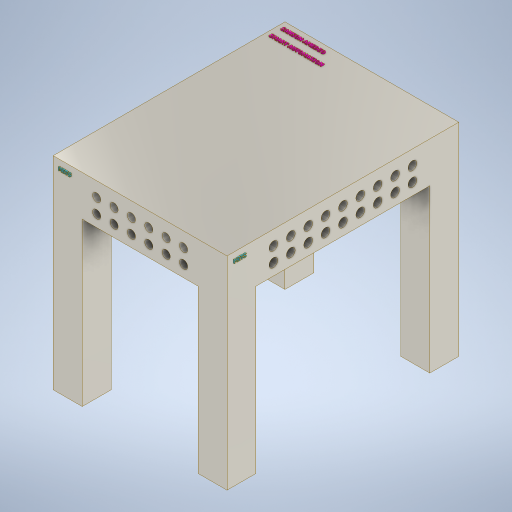
# Autodesk Inventor part: tavola d'appoggio 03-06-2023
Saved by Autodesk Inventor 2023 (Build 270158000, 158)
## iProperties
Created: 2023-03-06
Part Number: tavola d'appoggio 03-06-2023
Material: Generico
Document SubType Name: Modeling
Designer: Admin
Density: 1 g/cm^3
Appearance: Titanio
Author: Admin
Autodesk Inventor part; units mm, degrees
ref_plane "YZ Plane" through (0, 0, 0) normal (1, 0, 0) x (0, 1, 0)
ref_plane "XZ Plane" through (0, 0, 0) normal (0, 1, 0) x (-1, 0, 0)
ref_plane "XY Plane" through (0, 0, 0) normal (0, 0, 1) x (1, 0, 0)
sketch "Schizzo1" plane through (0, 0, 0) normal (0, 1, 0) x (-1, 0, 0)
  line L0 (150, 200) -> (-150, 200)
  line L1 (-150, 200) -> (-150, -200)
  line L2 (-150, -200) -> (150, -200)
  line L3 (150, -200) -> (150, 200)
  line L4 (150, 200) -> (100, 200)
  line L5 (100, 200) -> (100, 150)
  line L6 (100, 150) -> (150, 150)
  line L7 (-150, 200) -> (-150, 150)
  line L8 (-150, 150) -> (-100, 150)
  line L9 (-100, 150) -> (-100, 200)
  line L10 (-150, -200) -> (-150, -150)
  line L11 (-150, -150) -> (-100, -150)
  line L12 (-100, -150) -> (-100, -200)
  line L13 (150, -150) -> (100, -150)
  line L14 (100, -150) -> (100, -200)
  line L15 (125, -150) -> (125, 150)
  line L16 (100, 175) -> (-100, 175)
  line L17 (-125, 150) -> (-125, -150)
  line L18 (100, -175) -> (-100, -175)
  line L19 (0, 200) -> (0, -200) construction
  line L20 (150, 0) -> (-150, 0) construction
  point P0 (0, 0)
  dimension "d93" = 400
  dimension "d94" = 300
  dimension "d95" = 50
  constraints: 42 end point, 14 point on line, 12 midpoint, 7 perpendicular, 2 parallel, 1 horizontal, 1 horizontal alignment, 1 vertical, 1 vertical alignment, 3 other
  measures "d93" distance of L2.end L0.start
  measures "d94" distance of L0.start L0.end
  measures "d95" distance of L13.end L14.end
extrude "Estrusione5" add sketch "Schizzo1" along normal blind 350
extrude "Estrusione6" cut sketch "Schizzo1" along normal blind 340 contours L5 L6 L15 L13 L14 L18 L12 L11 L17 L8 L9 L16
extrude "Estrusione7" cut sketch "Schizzo1" along normal blind 280 contours L5 L16 L9 L0 | L3 L13 L15 L6 | L5 L6 L15 L13 L14 L18 L12 L11 L17 L8 L9 L16 | L8 L17 L11 L1 | L2 L12 L18 L14
sketch "Schizzo6" plane through (0, 0, 0) normal (1, 0, 0) x (0, 1, 0)
  circle A0 centre (325, 120) radius 7.5
  line L0 (340, -150) -> (340, 150) projected
  line L1 (0, 150) -> (340, 150) projected
  line L2 (340, 190) -> (340, 166.9269) construction
  line L3 (340, 166.9269) -> (300.9428, 166.9269) construction
  line L4 (300.9428, 166.9269) -> (300.9428, 190) construction
  line L5 (300.9428, 190) -> (340, 190) construction
  line L6 (0, 200) -> (350, 200) projected
  line L7 (350, -200) -> (350, 200) projected
  line L8 (333.7912, 183.1387) -> (333.7912, 184.6613)
  line L9 (333.7912, 184.6613) -> (337.8348, 184.6613)
  line L10 (337.8348, 184.6613) -> (335.2248, 185.7686)
  line L11 (335.2248, 185.7686) -> (335.2248, 186.8165)
  line L12 (335.2248, 186.8165) -> (337.8348, 187.9238)
  line L13 (337.8348, 187.9238) -> (333.7912, 187.9238)
  line L14 (333.7912, 187.9238) -> (333.7912, 189.3673)
  line L15 (333.7912, 189.3673) -> (339.8912, 189.3673)
  line L16 (339.8912, 189.3673) -> (339.8912, 187.6025)
  line L17 (339.8912, 187.6025) -> (336.8808, 186.2481)
  line L18 (336.8808, 186.2481) -> (339.8912, 184.9035)
  line L19 (339.8912, 184.9035) -> (339.8912, 183.1387)
  line L20 (339.8912, 183.1387) -> (333.7912, 183.1387)
  line L21 (333.7912, 178.8381) -> (333.7912, 182.1204)
  line L22 (333.7912, 182.1204) -> (334.8541, 182.1204)
  line L23 (334.8541, 182.1204) -> (334.8541, 181.2455)
  line L24 (334.8541, 181.2455) -> (338.8284, 181.2455)
  line L25 (338.8284, 181.2455) -> (338.8284, 182.1204)
  line L26 (338.8284, 182.1204) -> (339.8912, 182.1204)
  line L27 (339.8912, 182.1204) -> (339.8912, 178.8381)
  line L28 (339.8912, 178.8381) -> (338.8284, 178.8381)
  line L29 (338.8284, 178.8381) -> (338.8284, 179.713)
  line L30 (338.8284, 179.713) -> (334.8541, 179.713)
  line L31 (334.8541, 179.713) -> (334.8541, 178.8381)
  line L32 (334.8541, 178.8381) -> (333.7912, 178.8381)
  line L33 (333.7912, 176.6482) -> (338.7296, 176.6482)
  line L34 (338.7296, 176.6482) -> (338.7296, 178.4525)
  line L35 (338.7296, 178.4525) -> (339.8912, 178.4525)
  line L36 (339.8912, 178.4525) -> (339.8912, 173.3115)
  line L37 (339.8912, 173.3115) -> (338.7296, 173.3115)
  line L38 (338.7296, 173.3115) -> (338.7296, 175.1158)
  line L39 (338.7296, 175.1158) -> (333.7912, 175.1158)
  line L40 (333.7912, 175.1158) -> (333.7912, 176.6482)
  spline S0 degree 2 poles (333.6825, 170.8003) (333.6825, 171.5023) (333.9544, 172.5601) (334.1521, 173.0149) knots 0 0 0 1 2 2 2
  line L41 (334.1521, 173.0149) -> (335.6054, 173.0149)
  line L42 (335.6054, 173.0149) -> (335.6054, 172.8765)
  spline S1 degree 2 poles (335.6054, 172.8765) (335.2149, 172.4168) (334.7947, 171.3144) (334.7947, 170.7954) knots 0 0 0 1 2 2 2
  spline S2 degree 2 poles (334.7947, 170.7954) (334.7947, 170.6619) (334.8541, 170.2318) (334.9134, 170.1033) knots 0 0 0 1 2 2 2
  spline S3 degree 2 poles (334.9134, 170.1033) (334.9826, 169.9451) (335.2347, 169.7227) (335.4374, 169.7227) knots 0 0 0 1 2 2 2
  spline S4 degree 2 poles (335.4374, 169.7227) (335.6697, 169.7227) (335.9564, 170.0835) (336.0207, 170.3307) knots 0 0 0 1 2 2 2
  spline S5 degree 2 poles (336.0207, 170.3307) (336.1047, 170.6421) (336.2481, 171.349) (336.3568, 171.6605) knots 0 0 0 1 2 2 2
  spline S6 degree 2 poles (336.3568, 171.6605) (336.604, 172.3673) (337.4493, 172.9803) (338.082, 172.9803) knots 0 0 0 1 2 2 2
  spline S7 degree 2 poles (338.082, 172.9803) (338.9372, 172.9803) (340, 171.5319) (340, 170.4444) knots 0 0 0 1 2 2 2
  spline S8 degree 2 poles (340, 170.4444) (340, 169.9006) (339.7776, 168.823) (339.5897, 168.3979) knots 0 0 0 1 2 2 2
  line L43 (339.5897, 168.3979) -> (338.1957, 168.3979)
  line L44 (338.1957, 168.3979) -> (338.1957, 168.5314)
  spline S9 degree 2 poles (338.1957, 168.5314) (338.4874, 168.8724) (338.8878, 169.8512) (338.8878, 170.3653) knots 0 0 0 1 2 2 2
  spline S10 degree 2 poles (338.8878, 170.3653) (338.8878, 170.568) (338.8284, 170.8844) (338.7494, 171.0623) knots 0 0 0 1 2 2 2
  spline S11 degree 2 poles (338.7494, 171.0623) (338.6851, 171.2057) (338.428, 171.4133) (338.2699, 171.4133) knots 0 0 0 1 2 2 2
  spline S12 degree 2 poles (338.2699, 171.4133) (338.0326, 171.4133) (337.7607, 171.0821) (337.6519, 170.6075) knots 0 0 0 1 2 2 2
  spline S13 degree 2 poles (337.6519, 170.6075) (337.5827, 170.3011) (337.4493, 169.7326) (337.3356, 169.4063) knots 0 0 0 1 2 2 2
  spline S14 degree 2 poles (337.3356, 169.4063) (337.1032, 168.7736) (336.3321, 168.1557) (335.6994, 168.1557) knots 0 0 0 1 2 2 2
  spline S15 degree 2 poles (335.6994, 168.1557) (334.7898, 168.1557) (333.6825, 169.5843) (333.6825, 170.8003) knots 0 0 0 1 2 2 2
  point P0 (0, 0)
  dimension "d97" = 15
  dimension "d98" = 30
  dimension "d99" = 15
  dimension "d124" = 10
  dimension "d125" = 10
  constraints: 1 centre point, 2 other
  measures "d97" distance from line of L0 A0.centre
  measures "d98" distance from line of L1 A0.centre
  measures "d99" diameter of A0
  measures "d124" distance between parallel lines of L6 L5
  measures "d125" distance between parallel lines of L7 L2
extrude "Estrusione9" cut sketch "Schizzo6" along normal through all both and the other way through all contours A0
pattern_linear "Serie rettangolare1" count 9 spacing 30 along (0, 0, -1) count 2 spacing 25 along (0, -1, 0) of "Estrusione9"
sketch "Schizzo7" plane through (0, 0, 0) normal (0, 0, 1) x (1, 0, 0)
  circle A0 centre (-75, 325) radius 7.0059
  line L0 (-100, 0) -> (-100, 340) projected
  line L1 (-100, 280) -> (100, 280) projected
  line L2 (-140, 340) -> (-107.5524, 340) construction
  line L3 (-107.5524, 340) -> (-107.5524, 325.3132) construction
  line L4 (-107.5524, 325.3132) -> (-140, 325.3132) construction
  line L5 (-140, 325.3132) -> (-140, 340) construction
  line L6 (150, 350) -> (-150, 350) projected
  line L7 (-150, 0) -> (-150, 350) projected
  line L8 (-133.1387, 333.7912) -> (-134.6613, 333.7912)
  line L9 (-134.6613, 333.7912) -> (-134.6613, 337.8348)
  line L10 (-134.6613, 337.8348) -> (-135.7686, 335.2248)
  line L11 (-135.7686, 335.2248) -> (-136.8165, 335.2248)
  line L12 (-136.8165, 335.2248) -> (-137.9238, 337.8348)
  line L13 (-137.9238, 337.8348) -> (-137.9238, 333.7912)
  line L14 (-137.9238, 333.7912) -> (-139.3673, 333.7912)
  line L15 (-139.3673, 333.7912) -> (-139.3673, 339.8912)
  line L16 (-139.3673, 339.8912) -> (-137.6025, 339.8912)
  line L17 (-137.6025, 339.8912) -> (-136.2481, 336.8808)
  line L18 (-136.2481, 336.8808) -> (-134.9035, 339.8912)
  line L19 (-134.9035, 339.8912) -> (-133.1387, 339.8912)
  line L20 (-133.1387, 339.8912) -> (-133.1387, 333.7912)
  line L21 (-128.8381, 333.7912) -> (-132.1204, 333.7912)
  line L22 (-132.1204, 333.7912) -> (-132.1204, 334.8541)
  line L23 (-132.1204, 334.8541) -> (-131.2455, 334.8541)
  line L24 (-131.2455, 334.8541) -> (-131.2455, 338.8284)
  line L25 (-131.2455, 338.8284) -> (-132.1204, 338.8284)
  line L26 (-132.1204, 338.8284) -> (-132.1204, 339.8912)
  line L27 (-132.1204, 339.8912) -> (-128.8381, 339.8912)
  line L28 (-128.8381, 339.8912) -> (-128.8381, 338.8284)
  line L29 (-128.8381, 338.8284) -> (-129.713, 338.8284)
  line L30 (-129.713, 338.8284) -> (-129.713, 334.8541)
  line L31 (-129.713, 334.8541) -> (-128.8381, 334.8541)
  line L32 (-128.8381, 334.8541) -> (-128.8381, 333.7912)
  line L33 (-126.6482, 333.7912) -> (-126.6482, 338.7296)
  line L34 (-126.6482, 338.7296) -> (-128.4525, 338.7296)
  line L35 (-128.4525, 338.7296) -> (-128.4525, 339.8912)
  line L36 (-128.4525, 339.8912) -> (-123.3115, 339.8912)
  line L37 (-123.3115, 339.8912) -> (-123.3115, 338.7296)
  line L38 (-123.3115, 338.7296) -> (-125.1158, 338.7296)
  line L39 (-125.1158, 338.7296) -> (-125.1158, 333.7912)
  line L40 (-125.1158, 333.7912) -> (-126.6482, 333.7912)
  spline S0 degree 2 poles (-120.8003, 333.6825) (-121.5023, 333.6825) (-122.5601, 333.9544) (-123.0149, 334.1521) knots 0 0 0 1 2 2 2
  line L41 (-123.0149, 334.1521) -> (-123.0149, 335.6054)
  line L42 (-123.0149, 335.6054) -> (-122.8765, 335.6054)
  spline S1 degree 2 poles (-122.8765, 335.6054) (-122.4168, 335.2149) (-121.3144, 334.7947) (-120.7954, 334.7947) knots 0 0 0 1 2 2 2
  spline S2 degree 2 poles (-120.7954, 334.7947) (-120.6619, 334.7947) (-120.2318, 334.8541) (-120.1033, 334.9134) knots 0 0 0 1 2 2 2
  spline S3 degree 2 poles (-120.1033, 334.9134) (-119.9451, 334.9826) (-119.7227, 335.2347) (-119.7227, 335.4374) knots 0 0 0 1 2 2 2
  spline S4 degree 2 poles (-119.7227, 335.4374) (-119.7227, 335.6697) (-120.0835, 335.9564) (-120.3307, 336.0207) knots 0 0 0 1 2 2 2
  spline S5 degree 2 poles (-120.3307, 336.0207) (-120.6421, 336.1047) (-121.349, 336.2481) (-121.6605, 336.3568) knots 0 0 0 1 2 2 2
  spline S6 degree 2 poles (-121.6605, 336.3568) (-122.3673, 336.604) (-122.9803, 337.4493) (-122.9803, 338.082) knots 0 0 0 1 2 2 2
  spline S7 degree 2 poles (-122.9803, 338.082) (-122.9803, 338.9372) (-121.5319, 340) (-120.4444, 340) knots 0 0 0 1 2 2 2
  spline S8 degree 2 poles (-120.4444, 340) (-119.9006, 340) (-118.823, 339.7776) (-118.3979, 339.5897) knots 0 0 0 1 2 2 2
  line L43 (-118.3979, 339.5897) -> (-118.3979, 338.1957)
  line L44 (-118.3979, 338.1957) -> (-118.5314, 338.1957)
  spline S9 degree 2 poles (-118.5314, 338.1957) (-118.8724, 338.4874) (-119.8512, 338.8878) (-120.3653, 338.8878) knots 0 0 0 1 2 2 2
  spline S10 degree 2 poles (-120.3653, 338.8878) (-120.568, 338.8878) (-120.8844, 338.8284) (-121.0623, 338.7494) knots 0 0 0 1 2 2 2
  spline S11 degree 2 poles (-121.0623, 338.7494) (-121.2057, 338.6851) (-121.4133, 338.428) (-121.4133, 338.2699) knots 0 0 0 1 2 2 2
  spline S12 degree 2 poles (-121.4133, 338.2699) (-121.4133, 338.0326) (-121.0821, 337.7607) (-120.6075, 337.6519) knots 0 0 0 1 2 2 2
  spline S13 degree 2 poles (-120.6075, 337.6519) (-120.3011, 337.5827) (-119.7326, 337.4493) (-119.4063, 337.3356) knots 0 0 0 1 2 2 2
  spline S14 degree 2 poles (-119.4063, 337.3356) (-118.7736, 337.1032) (-118.1557, 336.3321) (-118.1557, 335.6994) knots 0 0 0 1 2 2 2
  spline S15 degree 2 poles (-118.1557, 335.6994) (-118.1557, 334.7898) (-119.5843, 333.6825) (-120.8003, 333.6825) knots 0 0 0 1 2 2 2
  point P0 (0, 0)
  dimension "d108" = 25
  dimension "d109" = 45
  dimension "d122" = 10
  dimension "d123" = 10
  constraints: 1 centre point, 2 other
  measures "d108" distance from line of L0 A0.centre
  measures "d109" distance from line of L1 A0.centre
  measures "d122" distance between parallel lines of L2 L6
  measures "d123" distance between parallel lines of L7 L5
extrude "Estrusione10" cut sketch "Schizzo7" along normal through all both and the other way through all contours A0
pattern_linear "Serie rettangolare2" count 6 spacing 30 along (1, 0, 0) count 2 spacing 25 along (0, -1, 0) of "Estrusione10"
sketch "Schizzo9" plane through (0, 350, 0) normal (0, 1, 0) x (1, 0, 0)
  line L0 (-142.233, 189.9265) -> (-17.7943, 189.9265) construction
  line L1 (-17.7943, 189.9265) -> (-17.7943, 153.1275) construction
  line L2 (-17.7943, 153.1275) -> (-142.233, 153.1275) construction
  line L3 (-142.233, 153.1275) -> (-142.233, 189.9265) construction
  spline S0 degree 2 poles (-139.7169, 183.5892) (-140.4189, 183.5892) (-141.4767, 183.8611) (-141.9315, 184.0588) knots 0 0 0 1 2 2 2
  line L4 (-141.9315, 184.0588) -> (-141.9315, 185.5122)
  line L5 (-141.9315, 185.5122) -> (-141.7931, 185.5122)
  spline S1 degree 2 poles (-141.7931, 185.5122) (-141.3334, 185.1217) (-140.231, 184.7015) (-139.712, 184.7015) knots 0 0 0 1 2 2 2
  spline S2 degree 2 poles (-139.712, 184.7015) (-139.5785, 184.7015) (-139.1484, 184.7608) (-139.0199, 184.8201) knots 0 0 0 1 2 2 2
  spline S3 degree 2 poles (-139.0199, 184.8201) (-138.8617, 184.8893) (-138.6393, 185.1414) (-138.6393, 185.3441) knots 0 0 0 1 2 2 2
  spline S4 degree 2 poles (-138.6393, 185.3441) (-138.6393, 185.5764) (-139.0001, 185.8631) (-139.2473, 185.9274) knots 0 0 0 1 2 2 2
  spline S5 degree 2 poles (-139.2473, 185.9274) (-139.5587, 186.0114) (-140.2656, 186.1548) (-140.5771, 186.2635) knots 0 0 0 1 2 2 2
  spline S6 degree 2 poles (-140.5771, 186.2635) (-141.2839, 186.5107) (-141.8969, 187.356) (-141.8969, 187.9888) knots 0 0 0 1 2 2 2
  spline S7 degree 2 poles (-141.8969, 187.9888) (-141.8969, 188.8439) (-140.4485, 189.9067) (-139.361, 189.9067) knots 0 0 0 1 2 2 2
  spline S8 degree 2 poles (-139.361, 189.9067) (-138.8172, 189.9067) (-137.7396, 189.6843) (-137.3145, 189.4965) knots 0 0 0 1 2 2 2
  line L6 (-137.3145, 189.4965) -> (-137.3145, 188.1024)
  line L7 (-137.3145, 188.1024) -> (-137.448, 188.1024)
  spline S9 degree 2 poles (-137.448, 188.1024) (-137.789, 188.3941) (-138.7678, 188.7945) (-139.2819, 188.7945) knots 0 0 0 1 2 2 2
  spline S10 degree 2 poles (-139.2819, 188.7945) (-139.4846, 188.7945) (-139.801, 188.7352) (-139.9789, 188.6561) knots 0 0 0 1 2 2 2
  spline S11 degree 2 poles (-139.9789, 188.6561) (-140.1223, 188.5918) (-140.3299, 188.3348) (-140.3299, 188.1766) knots 0 0 0 1 2 2 2
  spline S12 degree 2 poles (-140.3299, 188.1766) (-140.3299, 187.9393) (-139.9987, 187.6674) (-139.5241, 187.5587) knots 0 0 0 1 2 2 2
  spline S13 degree 2 poles (-139.5241, 187.5587) (-139.2177, 187.4895) (-138.6492, 187.356) (-138.3229, 187.2423) knots 0 0 0 1 2 2 2
  spline S14 degree 2 poles (-138.3229, 187.2423) (-137.6902, 187.01) (-137.0723, 186.2388) (-137.0723, 185.6061) knots 0 0 0 1 2 2 2
  spline S15 degree 2 poles (-137.0723, 185.6061) (-137.0723, 184.6965) (-138.5009, 183.5892) (-139.7169, 183.5892) knots 0 0 0 1 2 2 2
  line L8 (-136.9437, 183.698) -> (-134.8824, 189.798)
  line L9 (-134.8824, 189.798) -> (-133.2116, 189.798)
  line L10 (-133.2116, 189.798) -> (-131.1502, 183.698)
  line L11 (-131.1502, 183.698) -> (-132.7271, 183.698)
  line L12 (-132.7271, 183.698) -> (-133.1078, 184.9437)
  line L13 (-133.1078, 184.9437) -> (-135.0258, 184.9437)
  line L14 (-135.0258, 184.9437) -> (-135.4113, 183.698)
  line L15 (-135.4113, 183.698) -> (-136.9437, 183.698)
  line L16 (-133.4439, 186.051) -> (-134.0668, 188.0678)
  line L17 (-134.0668, 188.0678) -> (-134.6946, 186.051)
  line L18 (-134.6946, 186.051) -> (-133.4439, 186.051)
  line L19 (-125.3172, 183.698) -> (-126.7903, 183.698)
  line L20 (-126.7903, 183.698) -> (-129.1433, 187.9492)
  line L21 (-129.1433, 187.9492) -> (-129.1433, 183.698)
  line L22 (-129.1433, 183.698) -> (-130.5422, 183.698)
  line L23 (-130.5422, 183.698) -> (-130.5422, 189.798)
  line L24 (-130.5422, 189.798) -> (-128.6638, 189.798)
  line L25 (-128.6638, 189.798) -> (-126.7161, 186.3031)
  line L26 (-126.7161, 186.3031) -> (-126.7161, 189.798)
  line L27 (-126.7161, 189.798) -> (-125.3172, 189.798)
  line L28 (-125.3172, 189.798) -> (-125.3172, 183.698)
  spline S16 degree 2 poles (-122.193, 183.5892) (-122.895, 183.5892) (-123.9528, 183.8611) (-124.4076, 184.0588) knots 0 0 0 1 2 2 2
  line L29 (-124.4076, 184.0588) -> (-124.4076, 185.5122)
  line L30 (-124.4076, 185.5122) -> (-124.2692, 185.5122)
  spline S17 degree 2 poles (-124.2692, 185.5122) (-123.8095, 185.1217) (-122.7071, 184.7015) (-122.1881, 184.7015) knots 0 0 0 1 2 2 2
  spline S18 degree 2 poles (-122.1881, 184.7015) (-122.0546, 184.7015) (-121.6245, 184.7608) (-121.496, 184.8201) knots 0 0 0 1 2 2 2
  spline S19 degree 2 poles (-121.496, 184.8201) (-121.3378, 184.8893) (-121.1154, 185.1414) (-121.1154, 185.3441) knots 0 0 0 1 2 2 2
  spline S20 degree 2 poles (-121.1154, 185.3441) (-121.1154, 185.5764) (-121.4762, 185.8631) (-121.7234, 185.9274) knots 0 0 0 1 2 2 2
  spline S21 degree 2 poles (-121.7234, 185.9274) (-122.0348, 186.0114) (-122.7417, 186.1548) (-123.0531, 186.2635) knots 0 0 0 1 2 2 2
  spline S22 degree 2 poles (-123.0531, 186.2635) (-123.76, 186.5107) (-124.373, 187.356) (-124.373, 187.9888) knots 0 0 0 1 2 2 2
  spline S23 degree 2 poles (-124.373, 187.9888) (-124.373, 188.8439) (-122.9246, 189.9067) (-121.8371, 189.9067) knots 0 0 0 1 2 2 2
  spline S24 degree 2 poles (-121.8371, 189.9067) (-121.2933, 189.9067) (-120.2157, 189.6843) (-119.7906, 189.4965) knots 0 0 0 1 2 2 2
  line L31 (-119.7906, 189.4965) -> (-119.7906, 188.1024)
  line L32 (-119.7906, 188.1024) -> (-119.9241, 188.1024)
  spline S25 degree 2 poles (-119.9241, 188.1024) (-120.2651, 188.3941) (-121.2439, 188.7945) (-121.758, 188.7945) knots 0 0 0 1 2 2 2
  spline S26 degree 2 poles (-121.758, 188.7945) (-121.9607, 188.7945) (-122.2771, 188.7352) (-122.455, 188.6561) knots 0 0 0 1 2 2 2
  spline S27 degree 2 poles (-122.455, 188.6561) (-122.5984, 188.5918) (-122.806, 188.3348) (-122.806, 188.1766) knots 0 0 0 1 2 2 2
  spline S28 degree 2 poles (-122.806, 188.1766) (-122.806, 187.9393) (-122.4748, 187.6674) (-122.0002, 187.5587) knots 0 0 0 1 2 2 2
  spline S29 degree 2 poles (-122.0002, 187.5587) (-121.6937, 187.4895) (-121.1253, 187.356) (-120.799, 187.2423) knots 0 0 0 1 2 2 2
  spline S30 degree 2 poles (-120.799, 187.2423) (-120.1663, 187.01) (-119.5484, 186.2388) (-119.5484, 185.6061) knots 0 0 0 1 2 2 2
  spline S31 degree 2 poles (-119.5484, 185.6061) (-119.5484, 184.6965) (-120.977, 183.5892) (-122.193, 183.5892) knots 0 0 0 1 2 2 2
  spline S32 degree 2 poles (-113.2111, 186.748) (-113.2111, 185.265) (-114.7929, 183.5695) (-116.1672, 183.5695) knots 0 0 0 1 2 2 2
  spline S33 degree 2 poles (-116.1672, 183.5695) (-117.5463, 183.5695) (-119.1183, 185.2848) (-119.1183, 186.748) knots 0 0 0 1 2 2 2
  spline S34 degree 2 poles (-119.1183, 186.748) (-119.1183, 188.2161) (-117.5463, 189.9265) (-116.1672, 189.9265) knots 0 0 0 1 2 2 2
  spline S35 degree 2 poles (-116.1672, 189.9265) (-114.7929, 189.9265) (-113.2111, 188.226) (-113.2111, 186.748) knots 0 0 0 1 2 2 2
  spline S36 degree 2 poles (-114.7929, 186.748) (-114.7929, 187.2967) (-115.0154, 188.0629) (-115.2082, 188.3051) knots 0 0 0 1 2 2 2
  spline S37 degree 2 poles (-115.2082, 188.3051) (-115.401, 188.5572) (-115.8953, 188.7747) (-116.1622, 188.7747) knots 0 0 0 1 2 2 2
  spline S38 degree 2 poles (-116.1622, 188.7747) (-116.444, 188.7747) (-116.9037, 188.5721) (-117.1163, 188.315) knots 0 0 0 1 2 2 2
  spline S39 degree 2 poles (-117.1163, 188.315) (-117.3041, 188.0777) (-117.5365, 187.2918) (-117.5365, 186.748) knots 0 0 0 1 2 2 2
  spline S40 degree 2 poles (-117.5365, 186.748) (-117.5365, 186.1845) (-117.314, 185.443) (-117.1212, 185.1909) knots 0 0 0 1 2 2 2
  spline S41 degree 2 poles (-117.1212, 185.1909) (-116.9284, 184.9388) (-116.4292, 184.7212) (-116.1622, 184.7212) knots 0 0 0 1 2 2 2
  spline S42 degree 2 poles (-116.1622, 184.7212) (-115.8903, 184.7212) (-115.3861, 184.9536) (-115.2032, 185.2007) knots 0 0 0 1 2 2 2
  spline S43 degree 2 poles (-115.2032, 185.2007) (-115.0055, 185.4677) (-114.7929, 186.1746) (-114.7929, 186.748) knots 0 0 0 1 2 2 2
  line L33 (-107.0765, 183.698) -> (-108.5496, 183.698)
  line L34 (-108.5496, 183.698) -> (-110.9026, 187.9492)
  line L35 (-110.9026, 187.9492) -> (-110.9026, 183.698)
  line L36 (-110.9026, 183.698) -> (-112.3015, 183.698)
  line L37 (-112.3015, 183.698) -> (-112.3015, 189.798)
  line L38 (-112.3015, 189.798) -> (-110.4231, 189.798)
  line L39 (-110.4231, 189.798) -> (-108.4754, 186.3031)
  line L40 (-108.4754, 186.3031) -> (-108.4754, 189.798)
  line L41 (-108.4754, 189.798) -> (-107.0765, 189.798)
  line L42 (-107.0765, 189.798) -> (-107.0765, 183.698)
  line L43 (-104.0364, 183.698) -> (-101.975, 189.798)
  line L44 (-101.975, 189.798) -> (-100.3042, 189.798)
  line L45 (-100.3042, 189.798) -> (-98.2429, 183.698)
  line L46 (-98.2429, 183.698) -> (-99.8198, 183.698)
  line L47 (-99.8198, 183.698) -> (-100.2004, 184.9437)
  line L48 (-100.2004, 184.9437) -> (-102.1184, 184.9437)
  line L49 (-102.1184, 184.9437) -> (-102.504, 183.698)
  line L50 (-102.504, 183.698) -> (-104.0364, 183.698)
  line L51 (-100.5365, 186.051) -> (-101.1594, 188.0678)
  line L52 (-101.1594, 188.0678) -> (-101.7872, 186.051)
  line L53 (-101.7872, 186.051) -> (-100.5365, 186.051)
  line L54 (-91.4063, 183.698) -> (-92.9288, 183.698)
  line L55 (-92.9288, 183.698) -> (-92.9288, 187.7416)
  line L56 (-92.9288, 187.7416) -> (-94.0361, 185.1315)
  line L57 (-94.0361, 185.1315) -> (-95.0841, 185.1315)
  line L58 (-95.0841, 185.1315) -> (-96.1914, 187.7416)
  line L59 (-96.1914, 187.7416) -> (-96.1914, 183.698)
  line L60 (-96.1914, 183.698) -> (-97.6348, 183.698)
  line L61 (-97.6348, 183.698) -> (-97.6348, 189.798)
  line L62 (-97.6348, 189.798) -> (-95.8701, 189.798)
  line L63 (-95.8701, 189.798) -> (-94.5156, 186.7875)
  line L64 (-94.5156, 186.7875) -> (-93.1711, 189.798)
  line L65 (-93.1711, 189.798) -> (-91.4063, 189.798)
  line L66 (-91.4063, 189.798) -> (-91.4063, 183.698)
  line L67 (-90.1408, 183.698) -> (-90.1408, 189.798)
  line L68 (-90.1408, 189.798) -> (-86.0181, 189.798)
  line L69 (-86.0181, 189.798) -> (-86.0181, 188.6363)
  line L70 (-86.0181, 188.6363) -> (-88.6183, 188.6363)
  line L71 (-88.6183, 188.6363) -> (-88.6183, 187.5636)
  line L72 (-88.6183, 187.5636) -> (-86.2208, 187.5636)
  line L73 (-86.2208, 187.5636) -> (-86.2208, 186.402)
  line L74 (-86.2208, 186.402) -> (-88.6183, 186.402)
  line L75 (-88.6183, 186.402) -> (-88.6183, 184.8597)
  line L76 (-88.6183, 184.8597) -> (-86.0181, 184.8597)
  line L77 (-86.0181, 184.8597) -> (-86.0181, 183.698)
  line L78 (-86.0181, 183.698) -> (-90.1408, 183.698)
  spline S44 degree 2 poles (-79.5375, 186.743) (-79.5375, 185.8879) (-80.2839, 184.5433) (-80.8524, 184.1824) knots 0 0 0 1 2 2 2
  spline S45 degree 2 poles (-80.8524, 184.1824) (-81.327, 183.8759) (-82.4441, 183.698) (-83.0719, 183.698) knots 0 0 0 1 2 2 2
  line L79 (-83.0719, 183.698) -> (-84.98, 183.698)
  line L80 (-84.98, 183.698) -> (-84.98, 189.798)
  line L81 (-84.98, 189.798) -> (-83.0917, 189.798)
  spline S46 degree 2 poles (-83.0917, 189.798) (-82.4491, 189.798) (-81.327, 189.6349) (-80.8326, 189.3185) knots 0 0 0 1 2 2 2
  spline S47 degree 2 poles (-80.8326, 189.3185) (-80.2345, 188.9329) (-79.5375, 187.6279) (-79.5375, 186.743) knots 0 0 0 1 2 2 2
  spline S48 degree 2 poles (-81.1095, 186.7529) (-81.1095, 187.356) (-81.5247, 188.2161) (-81.9498, 188.4584) knots 0 0 0 1 2 2 2
  spline S49 degree 2 poles (-81.9498, 188.4584) (-82.2612, 188.6264) (-82.9434, 188.661) (-83.418, 188.661) knots 0 0 0 1 2 2 2
  line L82 (-83.418, 188.661) -> (-83.4476, 188.661)
  line L83 (-83.4476, 188.661) -> (-83.4476, 184.8399)
  line L84 (-83.4476, 184.8399) -> (-83.418, 184.8399)
  spline S50 degree 2 poles (-83.418, 184.8399) (-82.9039, 184.8399) (-82.197, 184.8745) (-81.8757, 185.0772) knots 0 0 0 1 2 2 2
  spline S51 degree 2 poles (-81.8757, 185.0772) (-81.5, 185.3144) (-81.1095, 186.1499) (-81.1095, 186.7529) knots 0 0 0 1 2 2 2
  line L85 (-78.6279, 183.698) -> (-78.6279, 189.798)
  line L86 (-78.6279, 189.798) -> (-74.5053, 189.798)
  line L87 (-74.5053, 189.798) -> (-74.5053, 188.6363)
  line L88 (-74.5053, 188.6363) -> (-77.1054, 188.6363)
  line L89 (-77.1054, 188.6363) -> (-77.1054, 187.5636)
  line L90 (-77.1054, 187.5636) -> (-74.7079, 187.5636)
  line L91 (-74.7079, 187.5636) -> (-74.7079, 186.402)
  line L92 (-74.7079, 186.402) -> (-77.1054, 186.402)
  line L93 (-77.1054, 186.402) -> (-77.1054, 184.8597)
  line L94 (-77.1054, 184.8597) -> (-74.5053, 184.8597)
  line L95 (-74.5053, 184.8597) -> (-74.5053, 183.698)
  line L96 (-74.5053, 183.698) -> (-78.6279, 183.698)
  spline S52 degree 2 poles (-67.9159, 186.748) (-67.9159, 185.265) (-69.4977, 183.5695) (-70.8719, 183.5695) knots 0 0 0 1 2 2 2
  spline S53 degree 2 poles (-70.8719, 183.5695) (-72.2511, 183.5695) (-73.8231, 185.2848) (-73.8231, 186.748) knots 0 0 0 1 2 2 2
  spline S54 degree 2 poles (-73.8231, 186.748) (-73.8231, 188.2161) (-72.2511, 189.9265) (-70.8719, 189.9265) knots 0 0 0 1 2 2 2
  spline S55 degree 2 poles (-70.8719, 189.9265) (-69.4977, 189.9265) (-67.9159, 188.226) (-67.9159, 186.748) knots 0 0 0 1 2 2 2
  spline S56 degree 2 poles (-69.4977, 186.748) (-69.4977, 187.2967) (-69.7202, 188.0629) (-69.9129, 188.3051) knots 0 0 0 1 2 2 2
  spline S57 degree 2 poles (-69.9129, 188.3051) (-70.1057, 188.5572) (-70.6001, 188.7747) (-70.867, 188.7747) knots 0 0 0 1 2 2 2
  spline S58 degree 2 poles (-70.867, 188.7747) (-71.1488, 188.7747) (-71.6085, 188.5721) (-71.8211, 188.315) knots 0 0 0 1 2 2 2
  spline S59 degree 2 poles (-71.8211, 188.315) (-72.0089, 188.0777) (-72.2412, 187.2918) (-72.2412, 186.748) knots 0 0 0 1 2 2 2
  spline S60 degree 2 poles (-72.2412, 186.748) (-72.2412, 186.1845) (-72.0188, 185.443) (-71.826, 185.1909) knots 0 0 0 1 2 2 2
  spline S61 degree 2 poles (-71.826, 185.1909) (-71.6332, 184.9388) (-71.1339, 184.7212) (-70.867, 184.7212) knots 0 0 0 1 2 2 2
  spline S62 degree 2 poles (-70.867, 184.7212) (-70.5951, 184.7212) (-70.0909, 184.9536) (-69.908, 185.2007) knots 0 0 0 1 2 2 2
  spline S63 degree 2 poles (-69.908, 185.2007) (-69.7103, 185.4677) (-69.4977, 186.1746) (-69.4977, 186.748) knots 0 0 0 1 2 2 2
  spline S64 degree 2 poles (-139.7169, 163.5023) (-140.4189, 163.5023) (-141.4767, 163.7741) (-141.9315, 163.9719) knots 0 0 0 1 2 2 2
  line L97 (-141.9315, 163.9719) -> (-141.9315, 165.4252)
  line L98 (-141.9315, 165.4252) -> (-141.7931, 165.4252)
  spline S65 degree 2 poles (-141.7931, 165.4252) (-141.3334, 165.0347) (-140.231, 164.6145) (-139.712, 164.6145) knots 0 0 0 1 2 2 2
  spline S66 degree 2 poles (-139.712, 164.6145) (-139.5785, 164.6145) (-139.1484, 164.6738) (-139.0199, 164.7331) knots 0 0 0 1 2 2 2
  spline S67 degree 2 poles (-139.0199, 164.7331) (-138.8617, 164.8023) (-138.6393, 165.0544) (-138.6393, 165.2571) knots 0 0 0 1 2 2 2
  spline S68 degree 2 poles (-138.6393, 165.2571) (-138.6393, 165.4895) (-139.0001, 165.7762) (-139.2473, 165.8404) knots 0 0 0 1 2 2 2
  spline S69 degree 2 poles (-139.2473, 165.8404) (-139.5587, 165.9245) (-140.2656, 166.0678) (-140.5771, 166.1766) knots 0 0 0 1 2 2 2
  spline S70 degree 2 poles (-140.5771, 166.1766) (-141.2839, 166.4237) (-141.8969, 167.269) (-141.8969, 167.9018) knots 0 0 0 1 2 2 2
  spline S71 degree 2 poles (-141.8969, 167.9018) (-141.8969, 168.757) (-140.4485, 169.8198) (-139.361, 169.8198) knots 0 0 0 1 2 2 2
  spline S72 degree 2 poles (-139.361, 169.8198) (-138.8172, 169.8198) (-137.7396, 169.5973) (-137.3145, 169.4095) knots 0 0 0 1 2 2 2
  line L99 (-137.3145, 169.4095) -> (-137.3145, 168.0155)
  line L100 (-137.3145, 168.0155) -> (-137.448, 168.0155)
  spline S73 degree 2 poles (-137.448, 168.0155) (-137.789, 168.3071) (-138.7678, 168.7075) (-139.2819, 168.7075) knots 0 0 0 1 2 2 2
  spline S74 degree 2 poles (-139.2819, 168.7075) (-139.4846, 168.7075) (-139.801, 168.6482) (-139.9789, 168.5691) knots 0 0 0 1 2 2 2
  spline S75 degree 2 poles (-139.9789, 168.5691) (-140.1223, 168.5049) (-140.3299, 168.2478) (-140.3299, 168.0896) knots 0 0 0 1 2 2 2
  spline S76 degree 2 poles (-140.3299, 168.0896) (-140.3299, 167.8523) (-139.9987, 167.5805) (-139.5241, 167.4717) knots 0 0 0 1 2 2 2
  spline S77 degree 2 poles (-139.5241, 167.4717) (-139.2177, 167.4025) (-138.6492, 167.269) (-138.3229, 167.1553) knots 0 0 0 1 2 2 2
  spline S78 degree 2 poles (-138.3229, 167.1553) (-137.6902, 166.923) (-137.0723, 166.1519) (-137.0723, 165.5191) knots 0 0 0 1 2 2 2
  spline S79 degree 2 poles (-137.0723, 165.5191) (-137.0723, 164.6096) (-138.5009, 163.5023) (-139.7169, 163.5023) knots 0 0 0 1 2 2 2
  line L101 (-130.0578, 163.611) -> (-131.5803, 163.611)
  line L102 (-131.5803, 163.611) -> (-131.5803, 167.6546)
  line L103 (-131.5803, 167.6546) -> (-132.6876, 165.0446)
  line L104 (-132.6876, 165.0446) -> (-133.7356, 165.0446)
  line L105 (-133.7356, 165.0446) -> (-134.8429, 167.6546)
  line L106 (-134.8429, 167.6546) -> (-134.8429, 163.611)
  line L107 (-134.8429, 163.611) -> (-136.2863, 163.611)
  line L108 (-136.2863, 163.611) -> (-136.2863, 169.711)
  line L109 (-136.2863, 169.711) -> (-134.5215, 169.711)
  line L110 (-134.5215, 169.711) -> (-133.1671, 166.7006)
  line L111 (-133.1671, 166.7006) -> (-131.8225, 169.711)
  line L112 (-131.8225, 169.711) -> (-130.0578, 169.711)
  line L113 (-130.0578, 169.711) -> (-130.0578, 163.611)
  line L114 (-129.4497, 163.611) -> (-127.3884, 169.711)
  line L115 (-127.3884, 169.711) -> (-125.7176, 169.711)
  line L116 (-125.7176, 169.711) -> (-123.6562, 163.611)
  line L117 (-123.6562, 163.611) -> (-125.2331, 163.611)
  line L118 (-125.2331, 163.611) -> (-125.6138, 164.8567)
  line L119 (-125.6138, 164.8567) -> (-127.5318, 164.8567)
  line L120 (-127.5318, 164.8567) -> (-127.9173, 163.611)
  line L121 (-127.9173, 163.611) -> (-129.4497, 163.611)
  line L122 (-125.9499, 165.964) -> (-126.5728, 167.9809)
  line L123 (-126.5728, 167.9809) -> (-127.2006, 165.964)
  line L124 (-127.2006, 165.964) -> (-125.9499, 165.964)
  line L125 (-117.4129, 163.611) -> (-119.2765, 163.611)
  line L126 (-119.2765, 163.611) -> (-120.972, 165.8503)
  line L127 (-120.972, 165.8503) -> (-121.5257, 165.8503)
  line L128 (-121.5257, 165.8503) -> (-121.5257, 163.611)
  line L129 (-121.5257, 163.611) -> (-123.0482, 163.611)
  line L130 (-123.0482, 163.611) -> (-123.0482, 169.711)
  line L131 (-123.0482, 169.711) -> (-120.5963, 169.711)
  spline S80 degree 2 poles (-120.5963, 169.711) (-120.0872, 169.711) (-119.3358, 169.5825) (-119.0145, 169.3848) knots 0 0 0 1 2 2 2
  spline S81 degree 2 poles (-119.0145, 169.3848) (-118.6882, 169.1771) (-118.3027, 168.5296) (-118.3027, 168.0352) knots 0 0 0 1 2 2 2
  spline S82 degree 2 poles (-118.3027, 168.0352) (-118.3027, 167.3382) (-118.9354, 166.4633) (-119.4643, 166.2062) knots 0 0 0 1 2 2 2
  line L132 (-119.4643, 166.2062) -> (-117.4129, 163.611)
  spline S83 degree 2 poles (-119.8746, 167.8425) (-119.8746, 168.0748) (-120.0526, 168.406) (-120.2553, 168.495) knots 0 0 0 1 2 2 2
  spline S84 degree 2 poles (-120.2553, 168.495) (-120.3986, 168.5543) (-120.7496, 168.5889) (-121.0116, 168.5889) knots 0 0 0 1 2 2 2
  line L133 (-121.0116, 168.5889) -> (-121.5257, 168.5889)
  line L134 (-121.5257, 168.5889) -> (-121.5257, 166.9477)
  line L135 (-121.5257, 166.9477) -> (-121.0857, 166.9477)
  spline S85 degree 2 poles (-121.0857, 166.9477) (-120.7694, 166.9477) (-120.3195, 167.0268) (-120.1663, 167.1504) knots 0 0 0 1 2 2 2
  spline S86 degree 2 poles (-120.1663, 167.1504) (-120.018, 167.269) (-119.8746, 167.5854) (-119.8746, 167.8425) knots 0 0 0 1 2 2 2
  line L136 (-115.7865, 163.611) -> (-115.7865, 168.5493)
  line L137 (-115.7865, 168.5493) -> (-117.5908, 168.5493)
  line L138 (-117.5908, 168.5493) -> (-117.5908, 169.711)
  line L139 (-117.5908, 169.711) -> (-112.4498, 169.711)
  line L140 (-112.4498, 169.711) -> (-112.4498, 168.5493)
  line L141 (-112.4498, 168.5493) -> (-114.2541, 168.5493)
  line L142 (-114.2541, 168.5493) -> (-114.2541, 163.611)
  line L143 (-114.2541, 163.611) -> (-115.7865, 163.611)
  line L144 (-110.0227, 163.611) -> (-107.9613, 169.711)
  line L145 (-107.9613, 169.711) -> (-106.2905, 169.711)
  line L146 (-106.2905, 169.711) -> (-104.2292, 163.611)
  line L147 (-104.2292, 163.611) -> (-105.8061, 163.611)
  line L148 (-105.8061, 163.611) -> (-106.1867, 164.8567)
  line L149 (-106.1867, 164.8567) -> (-108.1047, 164.8567)
  line L150 (-108.1047, 164.8567) -> (-108.4903, 163.611)
  line L151 (-108.4903, 163.611) -> (-110.0227, 163.611)
  line L152 (-106.5228, 165.964) -> (-107.1457, 167.9809)
  line L153 (-107.1457, 167.9809) -> (-107.7735, 165.964)
  line L154 (-107.7735, 165.964) -> (-106.5228, 165.964)
  spline S87 degree 2 poles (-101.1544, 163.4825) (-102.3853, 163.4825) (-103.7101, 164.6689) (-103.7101, 165.8157) knots 0 0 0 1 2 2 2
  line L155 (-103.7101, 165.8157) -> (-103.7101, 169.711)
  line L156 (-103.7101, 169.711) -> (-102.1777, 169.711)
  line L157 (-102.1777, 169.711) -> (-102.1777, 165.9047)
  spline S88 degree 2 poles (-102.1777, 165.9047) (-102.1777, 165.267) (-101.6982, 164.6442) (-101.1544, 164.6442) knots 0 0 0 1 2 2 2
  spline S89 degree 2 poles (-101.1544, 164.6442) (-100.6255, 164.6442) (-100.1312, 165.2423) (-100.1312, 165.9047) knots 0 0 0 1 2 2 2
  line L158 (-100.1312, 165.9047) -> (-100.1312, 169.711)
  line L159 (-100.1312, 169.711) -> (-98.5988, 169.711)
  line L160 (-98.5988, 169.711) -> (-98.5988, 165.8207)
  spline S90 degree 2 poles (-98.5988, 165.8207) (-98.5988, 164.6936) (-99.889, 163.4825) (-101.1544, 163.4825) knots 0 0 0 1 2 2 2
  line L161 (-96.2507, 163.611) -> (-96.2507, 168.5493)
  line L162 (-96.2507, 168.5493) -> (-98.055, 168.5493)
  line L163 (-98.055, 168.5493) -> (-98.055, 169.711)
  line L164 (-98.055, 169.711) -> (-92.914, 169.711)
  line L165 (-92.914, 169.711) -> (-92.914, 168.5493)
  line L166 (-92.914, 168.5493) -> (-94.7183, 168.5493)
  line L167 (-94.7183, 168.5493) -> (-94.7183, 163.611)
  line L168 (-94.7183, 163.611) -> (-96.2507, 163.611)
  spline S91 degree 2 poles (-86.7349, 166.661) (-86.7349, 165.178) (-88.3168, 163.4825) (-89.691, 163.4825) knots 0 0 0 1 2 2 2
  spline S92 degree 2 poles (-89.691, 163.4825) (-91.0702, 163.4825) (-92.6421, 165.1978) (-92.6421, 166.661) knots 0 0 0 1 2 2 2
  spline S93 degree 2 poles (-92.6421, 166.661) (-92.6421, 168.1292) (-91.0702, 169.8395) (-89.691, 169.8395) knots 0 0 0 1 2 2 2
  spline S94 degree 2 poles (-89.691, 169.8395) (-88.3168, 169.8395) (-86.7349, 168.139) (-86.7349, 166.661) knots 0 0 0 1 2 2 2
  spline S95 degree 2 poles (-88.3168, 166.661) (-88.3168, 167.2097) (-88.5392, 167.9759) (-88.732, 168.2181) knots 0 0 0 1 2 2 2
  spline S96 degree 2 poles (-88.732, 168.2181) (-88.9248, 168.4702) (-89.4191, 168.6878) (-89.686, 168.6878) knots 0 0 0 1 2 2 2
  spline S97 degree 2 poles (-89.686, 168.6878) (-89.9678, 168.6878) (-90.4275, 168.4851) (-90.6401, 168.228) knots 0 0 0 1 2 2 2
  spline S98 degree 2 poles (-90.6401, 168.228) (-90.8279, 167.9908) (-91.0603, 167.2048) (-91.0603, 166.661) knots 0 0 0 1 2 2 2
  spline S99 degree 2 poles (-91.0603, 166.661) (-91.0603, 166.0975) (-90.8378, 165.356) (-90.645, 165.1039) knots 0 0 0 1 2 2 2
  spline S100 degree 2 poles (-90.645, 165.1039) (-90.4523, 164.8518) (-89.953, 164.6343) (-89.686, 164.6343) knots 0 0 0 1 2 2 2
  spline S101 degree 2 poles (-89.686, 164.6343) (-89.4142, 164.6343) (-88.91, 164.8666) (-88.7271, 165.1138) knots 0 0 0 1 2 2 2
  spline S102 degree 2 poles (-88.7271, 165.1138) (-88.5293, 165.3807) (-88.3168, 166.0876) (-88.3168, 166.661) knots 0 0 0 1 2 2 2
  line L169 (-79.5968, 163.611) -> (-81.1194, 163.611)
  line L170 (-81.1194, 163.611) -> (-81.1194, 167.6546)
  line L171 (-81.1194, 167.6546) -> (-82.2266, 165.0446)
  line L172 (-82.2266, 165.0446) -> (-83.2746, 165.0446)
  line L173 (-83.2746, 165.0446) -> (-84.3819, 167.6546)
  line L174 (-84.3819, 167.6546) -> (-84.3819, 163.611)
  line L175 (-84.3819, 163.611) -> (-85.8253, 163.611)
  line L176 (-85.8253, 163.611) -> (-85.8253, 169.711)
  line L177 (-85.8253, 169.711) -> (-84.0606, 169.711)
  line L178 (-84.0606, 169.711) -> (-82.7061, 166.7006)
  line L179 (-82.7061, 166.7006) -> (-81.3616, 169.711)
  line L180 (-81.3616, 169.711) -> (-79.5968, 169.711)
  line L181 (-79.5968, 169.711) -> (-79.5968, 163.611)
  line L182 (-78.9888, 163.611) -> (-76.9275, 169.711)
  line L183 (-76.9275, 169.711) -> (-75.2566, 169.711)
  line L184 (-75.2566, 169.711) -> (-73.1953, 163.611)
  line L185 (-73.1953, 163.611) -> (-74.7722, 163.611)
  line L186 (-74.7722, 163.611) -> (-75.1528, 164.8567)
  line L187 (-75.1528, 164.8567) -> (-77.0708, 164.8567)
  line L188 (-77.0708, 164.8567) -> (-77.4564, 163.611)
  line L189 (-77.4564, 163.611) -> (-78.9888, 163.611)
  line L190 (-75.489, 165.964) -> (-76.1118, 167.9809)
  line L191 (-76.1118, 167.9809) -> (-76.7396, 165.964)
  line L192 (-76.7396, 165.964) -> (-75.489, 165.964)
  line L193 (-71.4157, 163.611) -> (-71.4157, 168.5493)
  line L194 (-71.4157, 168.5493) -> (-73.22, 168.5493)
  line L195 (-73.22, 168.5493) -> (-73.22, 169.711)
  line L196 (-73.22, 169.711) -> (-68.079, 169.711)
  line L197 (-68.079, 169.711) -> (-68.079, 168.5493)
  line L198 (-68.079, 168.5493) -> (-69.8833, 168.5493)
  line L199 (-69.8833, 168.5493) -> (-69.8833, 163.611)
  line L200 (-69.8833, 163.611) -> (-71.4157, 163.611)
  line L201 (-64.416, 163.611) -> (-67.6984, 163.611)
  line L202 (-67.6984, 163.611) -> (-67.6984, 164.6738)
  line L203 (-67.6984, 164.6738) -> (-66.8234, 164.6738)
  line L204 (-66.8234, 164.6738) -> (-66.8234, 168.6482)
  line L205 (-66.8234, 168.6482) -> (-67.6984, 168.6482)
  line L206 (-67.6984, 168.6482) -> (-67.6984, 169.711)
  line L207 (-67.6984, 169.711) -> (-64.416, 169.711)
  line L208 (-64.416, 169.711) -> (-64.416, 168.6482)
  line L209 (-64.416, 168.6482) -> (-65.291, 168.6482)
  line L210 (-65.291, 168.6482) -> (-65.291, 164.6738)
  line L211 (-65.291, 164.6738) -> (-64.416, 164.6738)
  line L212 (-64.416, 164.6738) -> (-64.416, 163.611)
  spline S103 degree 2 poles (-57.8464, 166.661) (-57.8464, 165.178) (-59.4283, 163.4825) (-60.8025, 163.4825) knots 0 0 0 1 2 2 2
  spline S104 degree 2 poles (-60.8025, 163.4825) (-62.1817, 163.4825) (-63.7536, 165.1978) (-63.7536, 166.661) knots 0 0 0 1 2 2 2
  spline S105 degree 2 poles (-63.7536, 166.661) (-63.7536, 168.1292) (-62.1817, 169.8395) (-60.8025, 169.8395) knots 0 0 0 1 2 2 2
  spline S106 degree 2 poles (-60.8025, 169.8395) (-59.4283, 169.8395) (-57.8464, 168.139) (-57.8464, 166.661) knots 0 0 0 1 2 2 2
  spline S107 degree 2 poles (-59.4283, 166.661) (-59.4283, 167.2097) (-59.6507, 167.9759) (-59.8435, 168.2181) knots 0 0 0 1 2 2 2
  spline S108 degree 2 poles (-59.8435, 168.2181) (-60.0363, 168.4702) (-60.5306, 168.6878) (-60.7976, 168.6878) knots 0 0 0 1 2 2 2
  spline S109 degree 2 poles (-60.7976, 168.6878) (-61.0793, 168.6878) (-61.539, 168.4851) (-61.7516, 168.228) knots 0 0 0 1 2 2 2
  spline S110 degree 2 poles (-61.7516, 168.228) (-61.9394, 167.9908) (-62.1718, 167.2048) (-62.1718, 166.661) knots 0 0 0 1 2 2 2
  spline S111 degree 2 poles (-62.1718, 166.661) (-62.1718, 166.0975) (-61.9493, 165.356) (-61.7565, 165.1039) knots 0 0 0 1 2 2 2
  spline S112 degree 2 poles (-61.7565, 165.1039) (-61.5638, 164.8518) (-61.0645, 164.6343) (-60.7976, 164.6343) knots 0 0 0 1 2 2 2
  spline S113 degree 2 poles (-60.7976, 164.6343) (-60.5257, 164.6343) (-60.0215, 164.8666) (-59.8386, 165.1138) knots 0 0 0 1 2 2 2
  spline S114 degree 2 poles (-59.8386, 165.1138) (-59.6408, 165.3807) (-59.4283, 166.0876) (-59.4283, 166.661) knots 0 0 0 1 2 2 2
  line L213 (-51.7118, 163.611) -> (-53.1849, 163.611)
  line L214 (-53.1849, 163.611) -> (-55.5379, 167.8622)
  line L215 (-55.5379, 167.8622) -> (-55.5379, 163.611)
  line L216 (-55.5379, 163.611) -> (-56.9369, 163.611)
  line L217 (-56.9369, 163.611) -> (-56.9369, 169.711)
  line L218 (-56.9369, 169.711) -> (-55.0584, 169.711)
  line L219 (-55.0584, 169.711) -> (-53.1108, 166.2161)
  line L220 (-53.1108, 166.2161) -> (-53.1108, 169.711)
  line L221 (-53.1108, 169.711) -> (-51.7118, 169.711)
  line L222 (-51.7118, 169.711) -> (-51.7118, 163.611)
  point P0 (0, 0)
  constraints: 2 other
extrude "Estrusione11" add sketch "Schizzo9" along normal blind 2
extrude "Estrusione12" add sketch "Schizzo6" along normal blind 152 contours L8 L9 L10 L11 L12 L13 L14 L15 L16 L17 L18 L19 L20 | L21 L22 L23 L24 L25 L26 L27 L28 L29 L30 L31 L32 | L33 L34 L35 L36 L37 L38 L39 L40 | S0 L41 L42 S1 S2 S3 S4 S5 S6 S7 S8 L43 L44 S9 S10 S11 S12 S13 S14 S15
extrude "Estrusione13" add sketch "Schizzo7" along normal blind 202 contours L8 L9 L10 L11 L12 L13 L14 L15 L16 L17 L18 L19 L20 | L21 L22 L23 L24 L25 L26 L27 L28 L29 L30 L31 L32 | L33 L34 L35 L36 L37 L38 L39 L40 | S0 L41 L42 S1 S2 S3 S4 S5 S6 S7 S8 L43 L44 S9 S10 S11 S12 S13 S14 S15
